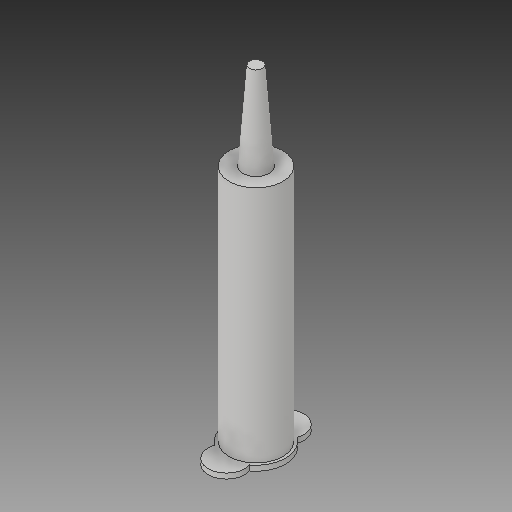
# Autodesk Inventor part: syringe
Saved by Autodesk Inventor 2018 (Build 220112000, 112)
## iProperties
Created: 2020-03-06
Part Number: syringe
Material: Generic
Document SubType Name: Modeling
Designer: Jesse R-B
Density: 1 g/cm^3
Appearance: Default
Author: Jesse R-B
Autodesk Inventor part; units mm, degrees
ref_plane "YZ Plane" through (0, 0, 0) normal (1, 0, 0) x (0, 1, 0)
ref_plane "XZ Plane" through (0, 0, 0) normal (0, 1, 0) x (-1, 0, 0)
sketch "Sketch1" plane through (0, 0, 0) normal (0, 1, 0) x (-1, 0, 0)
  circle A0 centre (0, 0) radius 10.4775
  dimension "d0" = 20.955
  constraints: 1 centre point, 1 coincident
  measures "d0" diameter of A0
extrude "Extrusion1" add sketch "Sketch1" along normal blind 95.25
sketch "Sketch2" plane through (0, 95.25, 0) normal (0, 1, 0) x (1, 0, 0)
  circle A0 centre (0, 0) radius 5.08
  dimension "d3" = 10.16
  constraints: 1 centre point, 1 coincident
  measures "d3" diameter of A0
ref_plane "Work Plane1" through (0, 129.54, 0) normal (0, 1, 0) x (1, 0, 0)
sketch "Sketch3" plane through (0, 129.54, 0) normal (0, 1, 0) x (1, 0, 0)
  circle A0 centre (0, 0) radius 2.54
  dimension "d5" = 5.08
  constraints: 1 centre point, 1 coincident
  measures "d5" diameter of A0
loft "Loft1" add profiles "Sketch2", "Sketch3"
sketch "Sketch4" plane through (0, 0, 0) normal (0, -1, 0) x (1, 0, 0)
  circle A0 centre (0, 0) radius 11.5507
  circle A1 centre (0, 11.5507) radius 7.1374
  circle A2 centre (0, -11.5507) radius 7.1374
  line L0 (7.1374, 11.5507) -> (11.5507, 0) construction
  line L1 (-7.1374, 11.5507) -> (-11.5507, 0) construction
  line L2 (-11.5507, 0) -> (-7.1374, -11.5507) construction
  line L3 (7.1374, -11.5507) -> (11.5507, 0) construction
  arc A3 (7.1374, 11.5507) -> (8.6078, 7.7021) centre (14.2137, 12.0492) ccw
  line L4 (11.5507, 0) -> (-11.5507, 0)
  line L5 (0, 11.5507) -> (0, -11.5507)
  arc A4 (-8.6078, 7.7021) -> (-7.1374, 11.5507) centre (-14.2137, 12.0492) ccw
  arc A5 (8.6078, -7.7021) -> (7.1374, -11.5507) centre (14.2137, -12.0492) ccw
  arc A6 (-7.1374, -11.5507) -> (-8.6078, -7.7021) centre (-14.2137, -12.0492) ccw
  circle A7 centre (0, 0) radius 11.5507
  dimension "d10" = 23.1013
  dimension "d11" = 14.2748
  dimension "d12" = 14.2748
  constraints: 18 point on circle, 12 end point, 8 centre point, 6 symmetric about line, 2 coincident, 1 concentric, 1 horizontal, 1 parallel, 1 perpendicular, 1 point on line, 3 other
  measures "d10" diameter of A0
  measures "d11" diameter of A1
  measures "d12" diameter of A2
extrude "Extrusion2" add sketch "Sketch4" against normal blind 2.032 contours L4 L5 A1 A0 | A0 A2 L5 L4 | L5 A2 A0 L4 | L4 A0 A1 L5 | A1 L5 A0 | A0 A1 | A2 A0 | A0 L5 A2 | A1 A0 L5 | L5 A0 A2
sketch "Sketch5" plane through (0, 0, 0) normal (0, -1, 0) x (1, 0, 0)
  circle A0 centre (0, 0) radius 5.08 projected
  circle A1 centre (0, 0) radius 9.6202
  dimension "d15" = 19.2405
  constraints: 1 centre point, 1 coincident
  measures "d15" diameter of A1
extrude "Extrusion3" cut sketch "Sketch5" against normal blind 93.5355 contours A0 | A1
body "Solid1"
